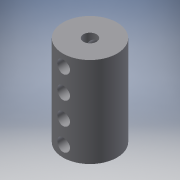
# Autodesk Inventor part: 00_Motorcoupling_5mm_M3
Saved by Autodesk Inventor 2019.4 (Build 234330000, 330)
## iProperties
Created: 2021-04-26
Part Number: 00_Motorcoupling_5mm_M3
Material: Generic
Document SubType Name: Modeling
Designer: diederichbenedict
Density: 1 g/cm^3
Appearance: Default
Author: diederichbenedict
Autodesk Inventor part; units mm, degrees
ref_plane "YZ Plane" through (0, 0, 0) normal (1, 0, 0) x (0, 1, 0)
ref_plane "XZ Plane" through (0, 0, 0) normal (0, 1, 0) x (-1, 0, 0)
ref_plane "XY Plane" through (0, 0, 0) normal (0, 0, 1) x (1, 0, 0)
sketch "Sketch1" plane through (0, 0, 0) normal (0, 1, 0) x (-1, 0, 0)
  circle A0 centre (0, 0) radius 6
  circle A1 centre (0, 0) radius 1.45
  dimension "d0" = 12
  dimension "d1" = 2.9
  constraints: 2 centre point, 2 coincident
  measures "d0" diameter of A0
  measures "d1" diameter of A1
extrude "Extrusion1" add sketch "Sketch1" along normal blind 20
sketch "Sketch2" plane through (0, 0, 0) normal (0, -1, 0) x (1, 0, 0)
  circle A0 centre (0, 0) radius 1.45 projected
  arc A1 (1.2894, -2.2) -> (-1.2894, -2.2) centre (0, 0) ccw
  line L0 (-1.2894, -2.2) -> (1.2894, -2.2)
  dimension "d4" = 5.1
  dimension "d5" = 2.2
  constraints: 2 end point, 2 point on circle, 1 centre point, 1 coincident, 1 horizontal
  measures "d4" diameter of A1
  measures "d5" distance from line of L0 point (0, 0)
extrude "Extrusion2" cut sketch "Sketch2" against normal blind 10
sketch "Sketch3" plane through (-1.2894, 0, -2.2) normal (0, 0, 1) x (1, 0, 0)
  line L0 (2.5788, 0) -> (2.5788, 10) projected
  line L1 (0, 0) -> (0, 10) projected
  circle A0 centre (1.2894, 2.469) radius 1.4
  point P0 (1.2894, 0)
  dimension "d8" = 2.8
  constraints: 1 centre point
  measures "d8" diameter of A0
extrude "Extrusion3" cut sketch "Sketch3" along normal mid plane 20
pattern_linear "Rectangular Pattern1" count 4 spacing 5 along (0, 1, 0) of "Extrusion3"
body "Solid1"
